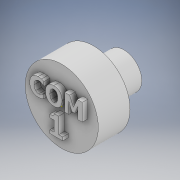
# Autodesk Inventor part: IPC Com 1 key
Saved by Autodesk Inventor 2022 (Build 260153000, 153)
## iProperties
Created: 2022-01-01
Part Number: IPC Com 1 key
Material: Generic
Document SubType Name: Modeling
Designer: solor
Density: 1 g/cm^3
Appearance: Default
Author: solor
Autodesk Inventor part; units mm, degrees
ref_plane "YZ Plane" through (0, 0, 0) normal (1, 0, 0) x (0, 1, 0)
ref_plane "XZ Plane" through (0, 0, 0) normal (0, 1, 0) x (-1, 0, 0)
ref_plane "XY Plane" through (0, 0, 0) normal (0, 0, 1) x (1, 0, 0)
sketch "Sketch1" plane through (0, 0, 0) normal (0, 0, 1) x (1, 0, 0)
  circle A0 centre (0, 0) radius 6.22 construction
  circle A1 centre (0, 0) radius 2.8
  line L0 (-0.675, 0.675) -> (-0.675, 2.025)
  line L1 (-0.675, 2.025) -> (0.675, 2.025)
  line L2 (0.675, 2.025) -> (0.675, 0.675)
  line L3 (0.675, 0.675) -> (2.025, 0.675)
  line L4 (2.025, 0.675) -> (2.025, -0.675)
  line L5 (2.025, -0.675) -> (0.675, -0.675)
  line L6 (0.675, -0.675) -> (0.675, -2.025)
  line L7 (0.675, -2.025) -> (-0.675, -2.025)
  line L8 (-0.675, -2.025) -> (-0.675, -0.675)
  line L9 (-0.675, -0.675) -> (-2.025, -0.675)
  line L10 (-2.025, -0.675) -> (-2.025, 0.675)
  line L11 (-2.025, 0.675) -> (-0.675, 0.675)
  circle A2 centre (0, 0) radius 5.75
  point P0 (-6.07, -6.1)
  dimension "d0" = 12.44
  dimension "d1" = 0.47
  constraints: 24 end point, 3 centre point, 1 coincident
  measures "d0" diameter of A0
  measures "d1" radial gap between concentric circles of A0 A2
extrude "Extrusion1" add sketch "Sketch1" along normal blind 5 contours A1 | L0 L1 L2 L3 L4 L5 L6 L7 L8 L9 L10 L11 | A2
extrude "Extrusion2" add sketch "Sketch1" against normal blind 4.8 contours A1
sketch "Sketch2" plane through (0, 0, 5) normal (0, 0, 1) x (1, 0, 0)
  point P0 (0, 0)
sketch "Sketch3" plane through (0, 0, 5) normal (0, 0, 1) x (1, 0, 0)
  line L0 (-4.2566, 3.1068) -> (4.2414, 3.1068) construction
  line L1 (4.2414, 3.1068) -> (4.2414, 0.2437) construction
  line L2 (4.2414, 0.2437) -> (-4.2566, 0.2437) construction
  line L3 (-4.2566, 0.2437) -> (-4.2566, 3.1068) construction
  line L4 (-1.3588, -0.6738) -> (1.3131, -0.6738) construction
  line L5 (1.3131, -0.6738) -> (1.3131, -3.7312) construction
  line L6 (1.3131, -3.7312) -> (-1.3588, -3.7312) construction
  line L7 (-1.3588, -3.7312) -> (-1.3588, -0.6738) construction
  spline S0 degree 2 poles (-2.8125, 0.2974) (-3.4208, 0.2974) (-4.1341, 1.0326) (-4.1341, 1.6977) knots 0 0 0 1 2 2 2
  spline S1 degree 2 poles (-4.1341, 1.6977) (-4.1341, 2.3388) (-3.4186, 3.1024) (-2.8103, 3.1024) knots 0 0 0 1 2 2 2
  spline S2 degree 2 poles (-2.8103, 3.1024) (-2.6506, 3.1024) (-2.3924, 3.0652) (-2.2743, 3.0346) knots 0 0 0 1 2 2 2
  spline S3 degree 2 poles (-2.2743, 3.0346) (-2.1824, 3.0062) (-1.9658, 2.9121) (-1.898, 2.8771) knots 0 0 0 1 2 2 2
  line L8 (-1.898, 2.8771) -> (-1.898, 2.2338)
  line L9 (-1.898, 2.2338) -> (-1.9658, 2.2338)
  spline S4 degree 2 poles (-1.9658, 2.2338) (-2.0161, 2.2775) (-2.1649, 2.4001) (-2.259, 2.457) knots 0 0 0 1 2 2 2
  spline S5 degree 2 poles (-2.259, 2.457) (-2.3531, 2.516) (-2.5784, 2.597) (-2.7031, 2.597) knots 0 0 0 1 2 2 2
  spline S6 degree 2 poles (-2.7031, 2.597) (-2.8497, 2.597) (-3.0926, 2.5051) (-3.2042, 2.3891) knots 0 0 0 1 2 2 2
  spline S7 degree 2 poles (-3.2042, 2.3891) (-3.3048, 2.2863) (-3.4339, 1.934) (-3.4339, 1.6955) knots 0 0 0 1 2 2 2
  spline S8 degree 2 poles (-3.4339, 1.6955) (-3.4339, 1.4439) (-3.3005, 1.1004) (-3.1911, 0.9954) knots 0 0 0 1 2 2 2
  spline S9 degree 2 poles (-3.1911, 0.9954) (-3.086, 0.8925) (-2.8279, 0.8028) (-2.6988, 0.8028) knots 0 0 0 1 2 2 2
  spline S10 degree 2 poles (-2.6988, 0.8028) (-2.5653, 0.8028) (-2.3224, 0.8925) (-2.2393, 0.9472) knots 0 0 0 1 2 2 2
  spline S11 degree 2 poles (-2.2393, 0.9472) (-2.1474, 1.0019) (-2.0095, 1.1179) (-1.9592, 1.1639) knots 0 0 0 1 2 2 2
  line L10 (-1.9592, 1.1639) -> (-1.898, 1.1639)
  line L11 (-1.898, 1.1639) -> (-1.898, 0.5293)
  spline S12 degree 2 poles (-1.898, 0.5293) (-1.9723, 0.4943) (-2.1671, 0.4068) (-2.2721, 0.3762) knots 0 0 0 1 2 2 2
  spline S13 degree 2 poles (-2.2721, 0.3762) (-2.399, 0.3368) (-2.62, 0.2974) (-2.8125, 0.2974) knots 0 0 0 1 2 2 2
  spline S14 degree 2 poles (0.9596, 1.6999) (0.9596, 1.0435) (0.2594, 0.293) (-0.3488, 0.293) knots 0 0 0 1 2 2 2
  spline S15 degree 2 poles (-0.3488, 0.293) (-0.9593, 0.293) (-1.6551, 1.0523) (-1.6551, 1.6999) knots 0 0 0 1 2 2 2
  spline S16 degree 2 poles (-1.6551, 1.6999) (-1.6551, 2.3498) (-0.9593, 3.1068) (-0.3488, 3.1068) knots 0 0 0 1 2 2 2
  spline S17 degree 2 poles (-0.3488, 3.1068) (0.2594, 3.1068) (0.9596, 2.3541) (0.9596, 1.6999) knots 0 0 0 1 2 2 2
  spline S18 degree 2 poles (0.2594, 1.6999) (0.2594, 1.9428) (0.161, 2.2819) (0.0756, 2.3891) knots 0 0 0 1 2 2 2
  spline S19 degree 2 poles (0.0756, 2.3891) (-0.0097, 2.5007) (-0.2285, 2.597) (-0.3467, 2.597) knots 0 0 0 1 2 2 2
  spline S20 degree 2 poles (-0.3467, 2.597) (-0.4714, 2.597) (-0.6749, 2.5073) (-0.7689, 2.3935) knots 0 0 0 1 2 2 2
  spline S21 degree 2 poles (-0.7689, 2.3935) (-0.8521, 2.2885) (-0.9549, 1.9406) (-0.9549, 1.6999) knots 0 0 0 1 2 2 2
  spline S22 degree 2 poles (-0.9549, 1.6999) (-0.9549, 1.4505) (-0.8565, 1.1223) (-0.7711, 1.0107) knots 0 0 0 1 2 2 2
  spline S23 degree 2 poles (-0.7711, 1.0107) (-0.6858, 0.8991) (-0.4648, 0.8028) (-0.3467, 0.8028) knots 0 0 0 1 2 2 2
  spline S24 degree 2 poles (-0.3467, 0.8028) (-0.2263, 0.8028) (-0.0031, 0.9057) (0.0778, 1.0151) knots 0 0 0 1 2 2 2
  spline S25 degree 2 poles (0.0778, 1.0151) (0.1653, 1.1332) (0.2594, 1.4461) (0.2594, 1.6999) knots 0 0 0 1 2 2 2
  line L12 (4.1191, 0.3499) -> (3.4452, 0.3499)
  line L13 (3.4452, 0.3499) -> (3.4452, 2.1397)
  line L14 (3.4452, 2.1397) -> (2.955, 0.9844)
  line L15 (2.955, 0.9844) -> (2.4912, 0.9844)
  line L16 (2.4912, 0.9844) -> (2.0011, 2.1397)
  line L17 (2.0011, 2.1397) -> (2.0011, 0.3499)
  line L18 (2.0011, 0.3499) -> (1.3622, 0.3499)
  line L19 (1.3622, 0.3499) -> (1.3622, 3.0499)
  line L20 (1.3622, 3.0499) -> (2.1433, 3.0499)
  line L21 (2.1433, 3.0499) -> (2.7428, 1.7174)
  line L22 (2.7428, 1.7174) -> (3.3379, 3.0499)
  line L23 (3.3379, 3.0499) -> (4.1191, 3.0499)
  line L24 (4.1191, 3.0499) -> (4.1191, 0.3499)
  line L25 (1.056, -3.7312) -> (-0.9584, -3.7312)
  line L26 (-0.9584, -3.7312) -> (-0.9584, -3.1998)
  line L27 (-0.9584, -3.1998) -> (-0.3157, -3.1998)
  line L28 (-0.3157, -3.1998) -> (-0.3157, -1.5858)
  line L29 (-0.3157, -1.5858) -> (-0.9584, -1.5858)
  line L30 (-0.9584, -1.5858) -> (-0.9584, -1.089)
  spline S26 degree 2 poles (-0.9584, -1.089) (-0.8175, -1.089) (-0.5382, -1.052) (-0.4541, -1.0124) knots 0 0 0 1 2 2 2
  spline S27 degree 2 poles (-0.4541, -1.0124) (-0.3578, -0.963) (-0.249, -0.7974) (-0.2391, -0.6738) knots 0 0 0 1 2 2 2
  line L31 (-0.2391, -0.6738) -> (0.4282, -0.6738)
  line L32 (0.4282, -0.6738) -> (0.4282, -3.1998)
  line L33 (0.4282, -3.1998) -> (1.056, -3.1998)
  line L34 (1.056, -3.1998) -> (1.056, -3.7312)
  point P0 (0, 0)
  point P1 (-0.0076, 0.2437)
  point P2 (-0.0228, -3.7312)
  constraints: 2 midpoint, 4 other
extrude "Extrusion3" add sketch "Sketch3" along normal blind 0.9
body "Solid1"
